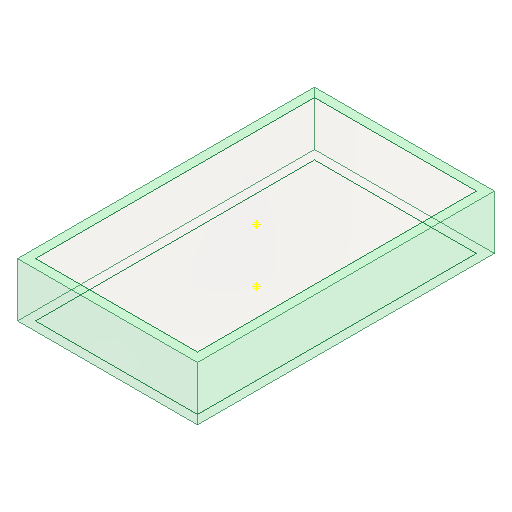
# Autodesk Inventor part: 3x4x1p2_KTN
Saved by Autodesk Inventor 2026.1 (Build 301233000, 233)
## iProperties
Created: 2022-10-15
Part Number: 3x4x1p2_KTN
Material: Generic
Document SubType Name: Modeling
Designer: kerlin
Density: 1 g/cm^3
Appearance: Default
Author: kerlin
Autodesk Inventor part; units mm, degrees
ref_plane "YZ Plane" through (0, 0, 0) normal (1, 0, 0) x (0, 1, 0)
ref_plane "XZ Plane" through (0, 0, 0) normal (0, 1, 0) x (-1, 0, 0)
ref_plane "XY Plane" through (0, 0, 0) normal (0, 0, 1) x (1, 0, 0)
sketch "Sketch1" plane through (0, 0, 0) normal (0, 1, 0) x (-1, 0, 0)
  line L0 (2, 3.3) -> (-2, 3.3)
  line L1 (-2, 3.3) -> (-2, -3.3)
  line L2 (-2, -3.3) -> (2, -3.3)
  line L3 (2, -3.3) -> (2, 3.3)
  line L4 (2, 3.3) -> (-2, -3.3) construction
  line L5 (-2, 3.3) -> (2, -3.3) construction
  point P0 (0, 0)
  dimension "d0" = 4
  dimension "d1" = 6.6
  constraints: 12 end point, 2 midpoint, 2 parallel, 1 horizontal, 1 perpendicular
  measures "d0" distance of L1.end L2.end
  measures "d1" distance of L0.end L1.end
extrude "Extrusion1" add sketch "Sketch1" along normal blind 1.2
sketch "Sketch2" plane through (0, 1.2, 0) normal (0, 1, 0) x (1, 0, 0)
  line L0 (-1.8, -3.1) -> (1.8, -3.1)
  line L1 (1.8, -3.1) -> (1.8, 3.1)
  line L2 (1.8, 3.1) -> (-1.8, 3.1)
  line L3 (-1.8, 3.1) -> (-1.8, -3.1)
  line L4 (-1.8, -3.1) -> (1.8, 3.1) construction
  line L5 (1.8, -3.1) -> (-1.8, 3.1) construction
  point P0 (0, 0)
  dimension "d4" = 3.6
  dimension "d5" = 6.2
  constraints: 12 end point, 2 midpoint, 2 parallel, 1 horizontal, 1 perpendicular
  measures "d4" distance of L1.end L2.end
  measures "d5" distance of L0.end L1.end
extrude "Extrusion2" add sketch "Sketch2" along normal blind 0.001
sketch "Sketch3" plane through (0, 0, 0) normal (0, -1, 0) x (1, 0, 0)
  line L0 (1.8, -3.1) -> (-1.8, -3.1)
  line L1 (-1.8, -3.1) -> (-1.8, 3.1)
  line L2 (-1.8, 3.1) -> (1.8, 3.1)
  line L3 (1.8, 3.1) -> (1.8, -3.1)
  line L4 (1.8, -3.1) -> (-1.8, 3.1) construction
  line L5 (-1.8, -3.1) -> (1.8, 3.1) construction
  point P0 (0, 0)
  dimension "d8" = 3.6
  dimension "d9" = 6.2
  constraints: 12 end point, 2 midpoint, 2 parallel, 1 horizontal, 1 perpendicular
  measures "d8" distance of L1.end L2.end
  measures "d9" distance of L0.end L1.end
extrude "Extrusion3" add sketch "Sketch3" along normal blind 0.001
body "Solid1"
